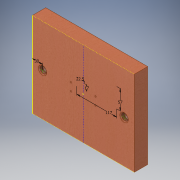
# Autodesk Inventor part: TablaInferior
Saved by Autodesk Inventor 2019 (Build 230136000, 136)
## iProperties
Created: 2019-05-15
Part Number: TablaInferior
Material: Generic
Document SubType Name: Modeling
Designer: Iván
Density: 1 g/cm^3
Appearance: Default
Author: Iván
Autodesk Inventor part; units mm, degrees
ref_plane "YZ Plane" through (0, 0, 0) normal (1, 0, 0) x (0, 1, 0)
ref_plane "XZ Plane" through (0, 0, 0) normal (0, 1, 0) x (-1, 0, 0)
ref_plane "XY Plane" through (0, 0, 0) normal (0, 0, 1) x (1, 0, 0)
sketch "Sketch1" plane through (0, 0, 0) normal (0, 0, 1) x (1, 0, 0)
  line L0 (-150, 125) -> (150, 125)
  line L1 (150, 125) -> (150, -125)
  line L2 (150, -125) -> (-150, -125)
  line L3 (-150, -125) -> (-150, 125)
  point P0 (0, 0)
  point P1 (0, 125)
  point P2 (150, 0)
  dimension "d0" = 300
  dimension "d1" = 250
  constraints: 8 end point, 2 midpoint, 2 parallel, 1 horizontal, 1 horizontal alignment, 1 perpendicular, 1 vertical alignment
  measures "d0" distance of L0.start L0.end
  measures "d1" distance of L0.end L1.end
extrude "Extrusion1" add sketch "Sketch1" along normal blind 39.37
sketch "Sketch2" plane through (0, 0, 39.37) normal (0, 0, 1) x (1, 0, 0)
  line L0 (-150, 125) -> (-150, -125) projected
  line L1 (150, 125) -> (-150, 125) construction
  line L2 (0, 125) -> (0, -125) construction
  line L3 (-150, -125) -> (150, -125) construction
  point P0 (0, 0)
  point P1 (-120, 0)
  point P2 (120, 0)
  dimension "d4" = 30
  constraints: 2 end point, 2 midpoint, 1 symmetric about line
  measures "d4" distance from line of L0 point (-120, 0)
hole "Hole1" at (-120, 0, 39.37) at (120, 0, 39.37) direction (0, 0, -1) diameter 10 end through all
hole "Hole2" at (-120, 0, 39.37) at (120, 0, 39.37) direction (0, 0, -1) diameter 20 depth 10 tip angle 118 countersink diameter 25 countersink angle 82
sketch "Sketch3" plane through (0, 0, 0) normal (0, 0, -1) x (-1, 0, 0)
  line L0 (58.5, -28.5) -> (-58.5, -28.5) construction
  line L1 (-58.5, -28.5) -> (-58.5, 28.5) construction
  line L2 (-58.5, 28.5) -> (58.5, 28.5) construction
  line L3 (58.5, 28.5) -> (58.5, -28.5) construction
  circle A0 centre (36, -11.5) radius 2
  line L4 (0, -28.5) -> (0, 28.5) construction
  line L5 (-58.5, 0) -> (58.5, 0) construction
  circle A1 centre (36, 11.5) radius 2
  circle A2 centre (-36, -11.5) radius 2
  circle A3 centre (-36, 11.5) radius 2
  point P0 (0, 0)
  dimension "d19" = 117
  dimension "d20" = 57
  dimension "d24" = 17
  dimension "d25" = 22.5
  constraints: 12 end point, 4 centre point, 4 midpoint, 3 symmetric about line, 2 parallel, 1 horizontal, 1 horizontal alignment, 1 perpendicular, 1 vertical alignment, 3 other
  measures "d19" distance of L0.start L0.end
  measures "d20" distance of L0.end L1.end
  measures "d24" distance from line of L0 A0.centre
  measures "d25" distance from line of L3 A0.centre
hole "Hole3" at (-36, -11.5, 0) at (-36, 11.5, 0) at (36, -11.5, 0) at (36, 11.5, 0) direction (0, 0, 1) diameter 4 end through all
hole "Hole4" at (36, 11.5, 0) at (36, -11.5, 0) at (-36, 11.5, 0) at (-36, -11.5, 0) direction (0, 0, 1) diameter 12 depth 8 tip angle 118
body "Solid1"
